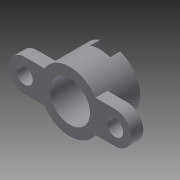
# Autodesk Inventor part: 零件1
Saved by Autodesk Inventor 2014 (Build 180170000, 170)
## iProperties
Created: 2018-11-23
Part Number: 零件1
Material: 常规
Document SubType Name: Modeling
Designer: Administrator
Density: 1 g/cm^3
Appearance: 默认
Author: Administrator
Autodesk Inventor part; units mm, degrees
ref_plane "YZ Plane" through (0, 0, 0) normal (1, 0, 0) x (0, 1, 0)
ref_plane "XZ Plane" through (0, 0, 0) normal (0, 1, 0) x (-1, 0, 0)
ref_plane "XY Plane" through (0, 0, 0) normal (0, 0, 1) x (1, 0, 0)
sketch "草图1" plane through (0, 0, 0) normal (0, 1, 0) x (-1, 0, 0)
  circle A0 centre (0, 0) radius 15
  circle A1 centre (0, 0) radius 10
  line L0 (0, 20.4744) -> (0, -21.3556)
  dimension "d0" = 30
  dimension "d1" = 20
  constraints: 2 centre point, 2 coincident, 2 end point, 1 vertical
  measures "d0" diameter of A0
  measures "d1" diameter of A1
extrude "拉伸1" add sketch "草图1" along normal blind 20 contours A0 L0 A1 | L0 A1 A0
sketch "草图2" plane through (0, 20, 0) normal (0, 1, 0) x (1, 0, 0)
  circle A0 centre (0, 0) radius 15 projected
  line L0 (-5, 17.5) -> (5, 17.5)
  line L1 (5, 17.5) -> (5, -17.5)
  line L2 (5, -17.5) -> (-5, -17.5)
  line L3 (-5, -17.5) -> (-5, 17.5)
  line L4 (-5, 17.5) -> (5, -17.5) construction
  line L5 (5, 17.5) -> (-5, -17.5) construction
  dimension "d5" = 10
  dimension "d6" = 35
  constraints: 12 end point, 2 midpoint, 2 parallel, 1 horizontal, 1 perpendicular
  measures "d5" distance of L1.end L2.end
  measures "d6" distance of L2.end L0.start
extrude "拉伸2" cut sketch "草图2" against normal blind 5 contours L1 A0 L3 | A0 L3 L0 L1 | L1 L2 L3 A0
sketch "草图3" plane through (0, 0, 0) normal (0, -1, 0) x (1, 0, 0)
  circle A0 centre (0, 0) radius 10 projected
  circle A1 centre (0, 0) radius 15 projected
  arc A2 (-22.5, 8) -> (-22.5, -8) centre (-22.5, 0) ccw
  line L0 (-22.5, 8) -> (-12.6886, 8)
  line L1 (-22.5, -8) -> (-12.6886, -8)
  circle A3 centre (22.5, 0) radius 4
  circle A4 centre (-22.5, 0) radius 4
  line L2 (0, 19.1751) -> (0, -20.0629)
  arc A5 (22.5, -8) -> (22.5, 8) centre (22.5, 0) ccw
  line L3 (22.5, 8) -> (12.6886, 8)
  line L4 (22.5, -8) -> (12.6886, -8)
  dimension "d10" = 16
  dimension "d11" = 8
  dimension "d12" = 16
  dimension "d13" = 45
  dimension "d14" = 22.5
  constraints: 10 end point, 8 point on circle, 4 centre point, 4 tangent, 2 coincident, 2 parallel, 2 perpendicular, 1 horizontal, 1 other
  measures "d10" diameter of A2
  measures "d11" diameter of A4
  measures "d12" diameter of A5
  measures "d13" distance of A3.centre A2.centre
  measures "d14" distance of A2.centre A0.centre
extrude "拉伸3" add sketch "草图3" against normal blind 6 contours L3 A5 L4 A1 | A1 L1 A2 L0
